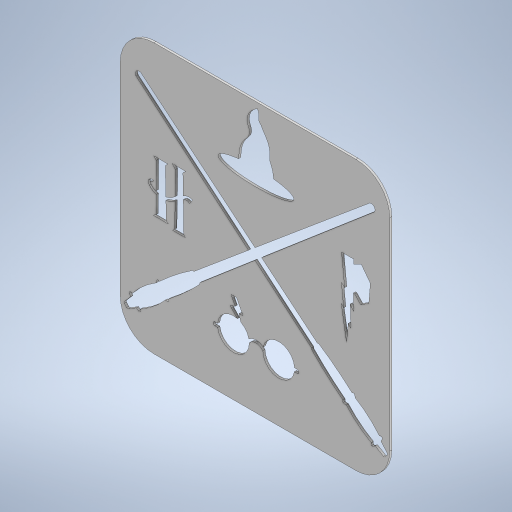
# Autodesk Inventor part: want cross sign panel
Saved by Autodesk Inventor 2024 (Build 280153000, 153)
## iProperties
Created: 2023-06-06
Part Number: want cross sign panel
Material: Generic
Document SubType Name: Modeling
Designer: newic
Density: 1 g/cm^3
Appearance: Default
Author: newic
Autodesk Inventor part; units mm, degrees
ref_plane "YZ Plane" through (0, 0, 0) normal (1, 0, 0) x (0, 1, 0)
ref_plane "XZ Plane" through (0, 0, 0) normal (0, 1, 0) x (-1, 0, 0)
ref_plane "XY Plane" through (0, 0, 0) normal (0, 0, 1) x (1, 0, 0)
sketch "Sketch1" plane through (0, 0, 0) normal (0, 0, 1) x (1, 0, 0)
  line L0 (50.8, 0) -> (355.6, 0)
  line L1 (406.4, 50.8) -> (406.4, 355.6)
  line L2 (355.6, 406.4) -> (50.8, 406.4)
  line L3 (0, 355.6) -> (0, 50.8)
  line L4 (-614.4193, 544.235) -> (888.7265, 544.235) construction
  line L5 (888.7265, 544.235) -> (888.7265, -583.1244) construction
  line L6 (888.7265, -583.1244) -> (-614.4193, -583.1244) construction
  line L7 (-614.4193, -583.1244) -> (-614.4193, 544.235) construction
  line L8 (6.3638, 43.7959) -> (9.7635, 39.8573)
  line L9 (12.1963, 39.4749) -> (24.4702, 46.9486)
  line L10 (24.4702, 46.9486) -> (27.5536, 44.5223)
  line L11 (29.7224, 44.3923) -> (30.075, 44.607)
  line L12 (30.938, 46.6729) -> (30.5528, 48.3003)
  arc A0 (30.5528, 48.3003) -> (68.0575, 78.8654) centre (-37.4709, 170.0608) ccw
  arc A1 (68.0575, 78.8654) -> (72.8989, 79.4068) centre (69.411, 88.6794) ccw
  arc A2 (72.8989, 79.4068) -> (72.8989, 82.7179) centre (67.458, 81.0624) ccw
  arc A3 (72.8989, 82.7179) -> (119.9382, 125.2394) centre (-186.4057, 416.8522) ccw
  arc A4 (119.9382, 125.2394) -> (119.9382, 127.3667) centre (115.2008, 126.3031) ccw
  arc A5 (383.5889, 351.7421) -> (376.4991, 359.9219) centre (378.6917, 354.66) ccw
  line L13 (6.3683, 46.2906) -> (15.8352, 57.179)
  line L14 (15.8352, 57.179) -> (13.9611, 60.6261)
  line L15 (14.1972, 62.7859) -> (14.4681, 63.0975)
  line L16 (16.6496, 63.6013) -> (18.1892, 62.9483)
  arc A6 (54.6184, 94.7874) -> (18.1892, 62.9483) centre (126.7971, -24.557) ccw
  arc A7 (55.9652, 99.4692) -> (54.6184, 94.7874) centre (64.5204, 94.4736) ccw
  arc A8 (59.2292, 98.9131) -> (55.9652, 99.4692) centre (56.6835, 93.8275) ccw
  arc A9 (109.0464, 138.1437) -> (59.2292, 98.9131) centre (345.0727, -212.821) ccw
  arc A10 (111.1434, 137.7865) -> (109.0464, 138.1437) centre (109.2993, 133.2949) ccw
  arc A11 (383.5352, 351.7378) -> (376.6079, 360.013) centre (378.6619, 354.6954) ccw
  arc A12 (27.5536, 44.5223) -> (29.7224, 44.3923) centre (28.7316, 46.0194) ccw
  arc A13 (9.7635, 39.8573) -> (12.1963, 39.4749) centre (11.2056, 41.102) ccw
  arc A14 (6.3683, 46.2906) -> (6.3638, 43.7959) centre (7.8059, 45.0407) ccw
  arc A15 (14.1972, 62.7859) -> (13.9611, 60.6261) centre (15.6348, 61.536) ccw
  arc A16 (16.6496, 63.6013) -> (14.4681, 63.0975) centre (15.9057, 61.8475) ccw
  arc A17 (30.075, 44.607) -> (30.938, 46.6729) centre (29.0843, 46.2341) ccw
  line L17 (399.5195, 39.8497) -> (402.8079, 43.8817)
  line L18 (402.762, 46.344) -> (393.2706, 57.1336)
  line L19 (393.2706, 57.1336) -> (395.1246, 60.5915)
  line L20 (394.876, 62.7499) -> (394.6033, 63.0599)
  line L21 (392.419, 63.551) -> (390.8831, 62.8891)
  arc A18 (390.8831, 62.8891) -> (354.2698, 94.5164) centre (282.7847, -25.2447) ccw
  arc A19 (354.2698, 94.5164) -> (352.8959, 99.1902) centre (344.3699, 94.1451) ccw
  arc A20 (352.8959, 99.1902) -> (349.6351, 98.6153) centre (352.2103, 93.5445) ccw
  arc A21 (349.6351, 98.6153) -> (299.5913, 137.5562) centre (65.6049, -214.7718) ccw
  arc A22 (299.5913, 137.5562) -> (297.4964, 137.1868) centre (299.3665, 132.706) ccw
  arc A23 (340.9233, 78.5167) -> (378.6047, 48.1697) centre (445.921, 170.3227) ccw
  line L22 (384.6951, 46.8533) -> (381.6258, 44.4091)
  line L23 (397.0619, 39.4209) -> (384.6951, 46.8533)
  line L24 (379.4578, 44.2665) -> (379.1039, 44.4792)
  line L25 (378.2289, 46.54) -> (378.6047, 48.1697)
  arc A24 (336.0788, 79.03) -> (340.9233, 78.5167) centre (339.5129, 88.3227) ccw
  arc A25 (336.0596, 82.341) -> (336.0788, 79.03) centre (341.5101, 80.7171) ccw
  arc A26 (288.7744, 124.589) -> (336.0596, 82.341) centre (593.4216, 417.9739) ccw
  arc A27 (288.7621, 126.7162) -> (288.7744, 124.589) centre (293.5057, 125.68) ccw
  arc A28 (30.8565, 357.7792) -> (23.8143, 349.5584) centre (28.6944, 352.5046) ccw
  arc A29 (395.1246, 60.5915) -> (394.876, 62.7499) centre (393.4457, 61.4916) ccw
  arc A30 (402.8079, 43.8817) -> (402.762, 46.344) centre (401.3317, 45.0857) ccw
  arc A31 (397.0619, 39.4209) -> (399.5195, 39.8497) centre (398.0432, 41.0538) ccw
  arc A32 (379.4578, 44.2665) -> (381.6258, 44.4091) centre (380.4391, 45.8993) ccw
  arc A33 (378.2289, 46.54) -> (379.1039, 44.4792) centre (380.0852, 46.112) ccw
  arc A34 (394.6033, 63.0599) -> (392.419, 63.551) centre (393.173, 61.8016) ccw
  line L26 (401.1476, 41.8459) -> (389.5741, 107.4826) construction
  line L27 (321.5532, 108.0825) -> (389.4683, 108.0825) construction
  circle A35 centre (170.7512, 85.86) radius 19.7773
  circle A36 centre (239.0957, 86.3674) radius 19.7773
  arc A37 (215.1665, 86.3674) -> (194.675, 86.3674) centre (204.9208, 78.7103) ccw
  arc A38 (215.6898, 91.3442) -> (194.0615, 91.2668) centre (204.9208, 78.7103) ccw
  line L28 (269.4046, 85.988) -> (269.4046, 84.6551)
  line L29 (140.6877, 84.6551) -> (140.6877, 85.988)
  line L30 (267.4996, 82.7501) -> (262.7499, 82.7501)
  line L31 (147.025, 82.7501) -> (142.5927, 82.7501)
  line L32 (142.5927, 87.893) -> (146.9086, 87.893)
  line L33 (262.9762, 87.893) -> (267.4996, 87.893)
  arc A39 (142.5927, 87.893) -> (140.6877, 85.988) centre (142.5927, 85.988) ccw
  arc A40 (140.6877, 84.6551) -> (142.5927, 82.7501) centre (142.5927, 84.6551) ccw
  arc A41 (267.4996, 82.7501) -> (269.4046, 84.6551) centre (267.4996, 84.6551) ccw
  arc A42 (269.4046, 85.988) -> (267.4996, 87.893) centre (267.4996, 85.988) ccw
  line L34 (176.8058, 109.0105) -> (165.9333, 120.456)
  line L35 (173.3684, 123.6889) -> (167.3787, 135.4678)
  line L36 (167.6051, 135.8369) -> (175.4776, 135.8369)
  line L37 (175.704, 135.6981) -> (185.0258, 117.3664)
  line L38 (184.7994, 116.9973) -> (179.6725, 116.9973)
  line L39 (179.426, 116.6819) -> (181.8153, 107.0777)
  line L40 (166.0352, 120.8712) -> (173.2243, 123.3335)
  arc A43 (166.0352, 120.8712) -> (165.9333, 120.456) centre (166.1175, 120.6309) ccw
  arc A44 (179.6725, 116.9973) -> (179.426, 116.6819) centre (179.6725, 116.7433) ccw
  arc A45 (173.2243, 123.3335) -> (173.3684, 123.6889) centre (173.142, 123.5737) ccw
  arc A46 (184.7994, 116.9973) -> (185.0258, 117.3664) centre (184.7994, 117.2513) ccw
  arc A47 (175.704, 135.6981) -> (175.4776, 135.8369) centre (175.4776, 135.5829) ccw
  arc A48 (167.6051, 135.8369) -> (167.3787, 135.4678) centre (167.6051, 135.5829) ccw
  line L41 (79.1785, 175.5287) -> (98.2166, 175.5287)
  line L42 (98.2166, 175.5287) -> (95.7577, 177.6666)
  line L43 (79.1785, 175.5287) -> (82.3225, 178.5153)
  line L44 (83.4016, 257.1181) -> (78.4147, 262.3678)
  line L45 (78.4147, 262.3678) -> (99.063, 262.3678)
  line L46 (99.063, 262.3678) -> (94.6597, 258.1849)
  arc A49 (104.8768, 223.4583) -> (95.1312, 223.6069) centre (99.9255, 218.3811) ccw
  arc A50 (103.2461, 231.2623) -> (95.0669, 228.3229) centre (103.7172, 217.1021) ccw
  arc A51 (109.0464, 230.1217) -> (103.2461, 231.2623) centre (102.6047, 212.6826) ccw
  line L47 (104.8768, 223.4583) -> (109.0464, 230.1217)
  arc A52 (68.9341, 213.9931) -> (82.9108, 221.3653) centre (58.8331, 250.0785) ccw
  arc A53 (69.0046, 209.415) -> (82.8332, 215.7132) centre (58.8331, 250.0785) ccw
  line L48 (68.3092, 254.5828) -> (71.9258, 258.4654)
  line L49 (71.9258, 258.4654) -> (50.44, 258.5979)
  line L50 (50.44, 258.5979) -> (54.6184, 254.7057)
  line L51 (54.1802, 183.6289) -> (50.217, 180.7223)
  line L52 (50.217, 180.7223) -> (72.4731, 180.5851)
  line L53 (72.4731, 180.5851) -> (69.411, 183.0161)
  arc A54 (49.8767, 216.0001) -> (54.3728, 214.8708) centre (53.3276, 220.2242) ccw
  arc A55 (46.1111, 220.5189) -> (49.8767, 216.0001) centre (54.3035, 223.5175) ccw
  arc A56 (46.5392, 223.6069) -> (46.1111, 220.5189) centre (48.4491, 221.7684) ccw
  arc A57 (49.3035, 223.7469) -> (46.5392, 223.6069) centre (48.0371, 221.3902) ccw
  arc A58 (50.4953, 225.8593) -> (49.3035, 223.7469) centre (51.8423, 223.7069) ccw
  arc A59 (50.4953, 225.8593) -> (46.5392, 226.3299) centre (48.1218, 222.7703) ccw
  arc A60 (46.5392, 226.3299) -> (42.6292, 222.9014) centre (48.7807, 219.8298) ccw
  arc A61 (42.6292, 222.9014) -> (44.2476, 216.9341) centre (48.1594, 221.1981) ccw
  arc A62 (44.2476, 216.9341) -> (54.3434, 210.1016) centre (58.2418, 226.7371) ccw
  ellipse E0 centre (204.8613, 307.5203) end of major axis (261.9878, 307.5203) minor radius 12.5901 (178.4242, 318.681) -> (231.2985, 318.681) ccw
  spline S0 degree 4 poles (178.4242, 318.681) (179.2865, 323.9088) (178.7469, 329.9031) (181.7055, 341.1617) (188.3746, 349.2769) (192.5951, 353.9732) (195.221, 358.5163) (195.2962, 364.6882) (192.6641, 369.2673) (190.583, 375.8582) (192.8313, 385.5671) (196.9449, 391.6863) (204.6887, 396.9503) (206.4239, 398.2659) knots 0 0 0 0 0 0.211951 0.294342 0.371604 0.443199 0.51143 0.580485 0.652609 0.727419 0.807137 1 1 1 1 1
  spline S1 degree 4 poles (231.2985, 318.681) (230.8123, 323.3837) (230.3106, 325.9488) (229.9675, 332.2974) (225.1644, 337.8653) (225.7946, 343.6095) (225.873, 348.5699) (225.5963, 353.1361) (224.2688, 359.1691) (219.9061, 368.5369) (215.481, 372.8733) (212.6971, 379.7041) (210.0846, 381.9551) (208.3589, 383.7283) (209.1642, 389.0307) (208.7268, 393.4813) (209.3508, 395.6633) (206.388, 397.7933) (206.4239, 398.2659) knots 0 0 0 0 0 0.148683 0.206661 0.265627 0.323445 0.38253 0.447581 0.516769 0.589023 0.656071 0.711518 0.763121 0.811155 0.858147 0.906117 1 1 1 1 1
  line L54 (344.0206, 186.4656) -> (341.2273, 160.6174)
  line L55 (341.2273, 160.6174) -> (333.4095, 207.3671)
  line L56 (333.4095, 207.3671) -> (336.9927, 203.1653)
  line L57 (336.9927, 203.1653) -> (333.6733, 234.7807)
  line L58 (333.6733, 234.7807) -> (338.5195, 230.3872)
  line L59 (338.5195, 230.3872) -> (333.8914, 274.4672)
  line L60 (333.8914, 274.4672) -> (352.2103, 274.4672)
  line L61 (352.2103, 274.4672) -> (352.2103, 267.6404)
  line L62 (352.2103, 267.6404) -> (363.5766, 273.4202)
  line L63 (363.5766, 273.4202) -> (377.295, 255.3431)
  line L64 (377.295, 255.3431) -> (374.9997, 227.9221)
  line L65 (374.9997, 227.9221) -> (362.5853, 220.2242)
  line L66 (362.5853, 220.2242) -> (353.7755, 229.6916)
  line L67 (353.7755, 229.6916) -> (351.6868, 229.9173)
  line L68 (351.6868, 229.9173) -> (352.0141, 205.912)
  line L69 (352.0141, 205.912) -> (346.9063, 213.1683)
  line L70 (346.9063, 213.1683) -> (347.8922, 181.9256)
  line L71 (347.8922, 181.9256) -> (344.0206, 186.4656)
  line L72 (351.6588, 231.9662) -> (353.6372, 231.7524)
  line L73 (353.6372, 231.7524) -> (359.5832, 227.5192)
  line L74 (359.5832, 227.5192) -> (362.1731, 227.1096)
  line L75 (362.1731, 227.1096) -> (364.2496, 230.6056)
  line L76 (364.2496, 230.6056) -> (362.5853, 266.6723)
  line L77 (362.5853, 266.6723) -> (352.0141, 262.7423)
  line L78 (352.0141, 262.7423) -> (351.6588, 231.9662)
  line L79 (94.6597, 258.1849) -> (95.0669, 228.3229)
  line L80 (95.1312, 223.6069) -> (95.7577, 177.6666)
  line L81 (82.3225, 178.5153) -> (82.8332, 215.7132)
  line L82 (82.9108, 221.3653) -> (83.4016, 257.1181)
  line L83 (69.411, 183.0161) -> (69.0046, 209.415)
  line L84 (68.9341, 213.9931) -> (68.3092, 254.5828)
  line L85 (54.6184, 254.7057) -> (54.3728, 214.8708)
  line L86 (54.3434, 210.1016) -> (54.1802, 183.6289)
  line L87 (288.7621, 126.7162) -> (203.4692, 198.4543)
  line L88 (193.5656, 206.784) -> (23.8143, 349.5584)
  line L89 (111.1434, 137.7865) -> (193.5656, 206.784)
  line L90 (203.4099, 215.0249) -> (376.6079, 360.013)
  line L91 (297.4964, 137.1868) -> (213.3132, 206.8319)
  line L92 (203.4099, 215.0249) -> (30.7472, 357.8696)
  line L93 (119.9382, 127.3667) -> (203.4692, 198.4543)
  line L94 (213.3132, 206.8319) -> (383.5889, 351.7421)
  arc A63 (147.025, 82.7501) -> (194.675, 86.3674) centre (170.7512, 85.86) ccw
  arc A64 (194.0615, 91.2668) -> (181.8153, 107.0777) centre (170.7512, 85.86) ccw
  arc A65 (176.8058, 109.0105) -> (146.9086, 87.893) centre (170.7512, 85.86) ccw
  arc A66 (215.1665, 86.3674) -> (262.7499, 82.7501) centre (239.0957, 86.3674) ccw
  arc A67 (262.9762, 87.893) -> (215.6898, 91.3442) centre (239.0957, 86.3674) ccw
  arc A68 (0, 50.8) -> (50.8, 0) centre (50.8, 50.8) ccw
  arc A69 (355.6, 0) -> (406.4, 50.8) centre (355.6, 50.8) ccw
  arc A70 (406.4, 355.6) -> (355.6, 406.4) centre (355.6, 355.6) ccw
  arc A71 (50.8, 406.4) -> (0, 355.6) centre (50.8, 355.6) ccw
  point P0 (0, 0)
  point P1 (406.4, 406.4)
  point P2 (406.4, 0)
  point P3 (0, 406.4)
  point P4 (0, 51.1687)
  point P5 (10.818, 38.6356)
  point P6 (28.5929, 43.7045)
  point P7 (31.2567, 45.3266)
  point P8 (5.3476, 45.1167)
  point P9 (13.3295, 61.7879)
  point P10 (15.3759, 64.1415)
  point P11 (179.1982, 326.399)
  point P12 (180.6435, 334.8413)
  point P13 (184.2943, 343.588)
  point P14 (188.8575, 349.7483)
  point P15 (192.5838, 354.3872)
  point P16 (194.7132, 358.874)
  point P17 (194.7892, 364.1974)
  point P18 (192.9635, 369.2156)
  point P19 (191.3661, 375.5272)
  point P20 (192.431, 382.4481)
  point P21 (195.7774, 388.7607)
  point P22 (202.0895, 394.9967)
  point P23 (230.5589, 324.7909)
  point P24 (229.8649, 328.855)
  point P25 (228.2789, 333.5142)
  point P26 (225.9991, 338.1735)
  point P27 (225.7017, 343.6254)
  point P28 (225.8006, 348.3832)
  point P29 (225.5031, 352.5463)
  point P30 (224.1154, 358.4942)
  point P31 (219.5559, 368.0113)
  point P32 (215.0954, 374.5543)
  point P33 (211.9235, 380.0068)
  point P34 (210.0401, 382.0886)
  point P35 (208.9497, 383.9719)
  point P36 (208.9495, 388.928)
  point P37 (208.9493, 392.7935)
  point P38 (208.6516, 395.073)
  point P39 (207.1647, 397.2538)
  point P40 (383.033, 358.3545)
  dimension "d0" = 406.4
  dimension "d1" = 406.4
  dimension "d37" = 1.905
  dimension "d38" = 1.905
  dimension "d40" = 1.905
  dimension "d41" = 1.905
  dimension "d43" = 1.905
  dimension "d44" = 1.905
  dimension "d45" = 1.905
  dimension "d46" = 1.905
  dimension "d62" = 3.81
  dimension "d69" = 1.905
  dimension "d73" = 0.254
  dimension "d80" = 50.8
  constraints: 182 end point, 141 point on circle, 72 centre point, 52 tangent, 27 point on line, 15 equal radius, 15 parallel, 9 horizontal, 7 perpendicular, 2 coincident, 41 other
  measures "d0" distance of point (0, 406.4) point (406.4, 406.4)
  measures "d1" distance of point (406.4, 406.4) point (406.4, 0)
  measures "d37" radius of A12
  measures "d38" radius of A13
  measures "d40" radius of A14
  measures "d41" radius of A15
  measures "d43" radius of A29
  measures "d44" radius of A30
  measures "d45" radius of A31
  measures "d46" radius of A32
  measures "d62" radial gap between concentric circles of A37 A38
  measures "d69" radius of A39
  measures "d73" radius of A43
  measures "d80" radius of A68
extrude "Extrusion1" add sketch "Sketch1" along normal blind 3.175 contours A68 L3 A71 L2 A70 L1 A69 L0
body "Solid1"
